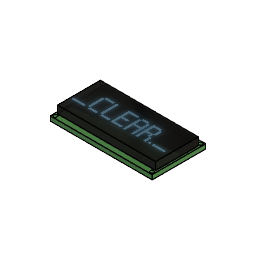
Screen approximate v5 (Autodesk Fusion 360 design; units mm, degrees)
Autodesk Fusion 360 part; units mm, degrees
box "BoxPrimitive1" add length 35 width 66.5 height 3 placed x (0, 1, 0) y (-1, 0, 0) z (0, 0, 1) at (66.4952, 0, 0) makes body 1
sketch "Sketch3" plane through (0, 0, 3) normal (0, 0, 1) x (-1, 0, 0)
  line L0 (-66.4952, -35) -> (0.0048, -35)
  line L1 (0.0048, -35) -> (0.0048, 0)
  line L2 (0.0048, 0) -> (-66.4952, 0)
  line L3 (-66.4952, 0) -> (-66.4952, -35)
  line L4 (0.0048, 0) -> (-66.4952, -35) construction
  line L5 (0.0048, -35) -> (-66.4952, 0) construction
  circle A0 centre (-1.6952, -33.3) radius 1.2
  line L6 (-33.2452, -17.5) -> (0.0048, -17.5) construction
  line L7 (-33.2452, -17.5) -> (-33.2452, -35) construction
  circle A1 centre (-1.6952, -1.7) radius 1.2
  circle A2 centre (-64.7952, -33.3) radius 1.2
  circle A3 centre (-64.7952, -1.7) radius 1.2
  line L8 (-65.2452, -3.5) -> (-1.2452, -3.5)
  line L9 (-1.2452, -3.5) -> (-1.2452, -31.5)
  line L10 (-1.2452, -31.5) -> (-65.2452, -31.5)
  line L11 (-65.2452, -31.5) -> (-65.2452, -3.5)
  line L12 (-65.2452, -3.5) -> (-1.2452, -31.5) construction
  line L13 (-1.2452, -3.5) -> (-65.2452, -31.5) construction
  point P0 (-33.2452, -17.5)
  dimension "d6" = 2.4
  dimension "d7" = 1.7
  dimension "d8" = 1.7
  dimension "d13" = 64
  dimension "d14" = 28
  constraint coincident L1.end L2.start
  constraint coincident L0.start L3.end
  constraint coincident L0.end L1.start
  constraint coincident L2.end L3.start
  constraint midpoint L4 P0
  constraint midpoint L1 L6.end
  constraint midpoint L0 L7.end
  constraint symmetric A0 L6 A1
  constraint symmetric A0 L7 A2
  constraint symmetric L7 A1 A3
  constraint horizontal L8
  constraint perpendicular L8 L9
  constraint parallel L8 L10
  constraint parallel L9 L11
  constraint coincident L12 P0
  constraint coincident L13 P0
  constraint coincident P0 L6.start
  measures "d6" diameter of A0
  measures "d7" distance of L1 A0.centre
  measures "d8" distance of L0 A0.centre
  measures "d13" distance of L8.start L8.end
  measures "d14" distance of L8.start L10.end
extrude "Extrude1" cut sketch "Sketch3" against normal through all contours A0 | A1 | A2 | A3 bodies 1
extrude "Extrude2" add sketch "Sketch3" along normal blind 5 separate body contours L8 L9 L10 L11 makes body 2
